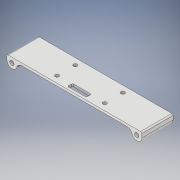
# Autodesk Inventor part: US Halterung hinten leicht
Saved by Autodesk Inventor 2018 (Build 220112000, 112)
## iProperties
Created: 2019-03-05
Part Number: US Halterung hinten leicht
Material: ABS-Kunststoff
Document SubType Name: Modeling
Designer: RedBots
Density: 0.732517 g/cm^3
Appearance: Glatt - weiß
Mass: 4 g
Surface Area: 43.527 cm^2
Volume: 5.46063 cm^3
Author: RedBots
Autodesk Inventor part; units mm, degrees
ref_plane "YZ Plane" through (0, 0, 0) normal (1, 0, 0) x (0, 1, 0)
ref_plane "XZ Plane" through (0, 0, 0) normal (0, 1, 0) x (-1, 0, 0)
ref_plane "XY Plane" through (0, 0, 0) normal (0, 0, 1) x (1, 0, 0)
sketch "Skizze1" plane through (0, 0, 0) normal (0, 0, 1) x (1, 0, 0)
  line L0 (0, 0) -> (108, 0)
  line L1 (108, 0) -> (108, 25)
  line L2 (108, 25) -> (0, 25)
  line L3 (0, 25) -> (0, 0)
  dimension "d5" = 108
  dimension "d6" = 25
  constraints: 8 end point, 2 parallel, 1 horizontal, 1 perpendicular
  measures "d5" distance of L1.end L2.end
  measures "d6" distance of L0.end L1.end
extrude "Extrusion1" add sketch "Skizze1" along normal blind 2
sketch "Skizze3" plane through (0, 25, 0) normal (0, 1, 0) x (1, 0, 0)
  circle A0 centre (4, 2) radius 1.75
  circle A1 centre (104, 2) radius 1.75
  line L0 (4, 2) -> (104, 2) construction
  line L1 (0, 0) -> (108, 0) construction
  line L2 (54, 0) -> (54, 2) construction
  line L3 (0, 0) -> (8, 0)
  line L4 (108, 0) -> (100, 0)
  line L5 (0, 0) -> (0, 2)
  line L6 (8, 2) -> (8, 0)
  line L7 (100, 2) -> (100, 0)
  line L8 (108, 0) -> (108, 2)
  arc A2 (8, 2) -> (0, 2) centre (4, 2) ccw
  arc A3 (108, 2) -> (100, 2) centre (104, 2) ccw
  dimension "d2" = 100
  dimension "d3" = 3.5
  dimension "d4" = 2
  constraints: 16 end point, 5 parallel, 4 centre point, 4 point on circle, 3 horizontal, 3 vertical, 2 coincident, 2 midpoint, 2 point on line, 1 equal radius
  measures "d2" distance of L0.start L0.end
  measures "d3" diameter of A0
  measures "d4" distance of L2.start L2.end
extrude "Extrusion2" add sketch "Skizze3" against normal up to surface (25 mm away)
sketch "Skizze4" plane through (0, 0, 2) normal (0, 0, 1) x (1, 0, 0)
  line L0 (34.95, 5.261) -> (73.05, 5.261) construction
  line L1 (73.05, 5.261) -> (73.05, 19.739) construction
  line L2 (73.05, 19.739) -> (34.95, 19.739) construction
  line L3 (34.95, 19.739) -> (34.95, 5.261) construction
  line L4 (108, 25) -> (0, 25) construction
  line L5 (54, 25) -> (54, 0) construction
  line L6 (0, 0) -> (108, 0) construction
  line L7 (0, 25) -> (0, 0) construction
  line L8 (0, 12.5) -> (108, 12.5) construction
  line L9 (108, 0) -> (108, 25) construction
  circle A0 centre (73.05, 19.739) radius 1.5
  circle A1 centre (34.95, 5.261) radius 1.5
  circle A2 centre (34.95, 19.739) radius 1.5
  circle A3 centre (73.05, 5.261) radius 1.5
  point P0 (54, 19.739)
  point P1 (73.05, 12.5)
  dimension "d12" = 38.1
  dimension "d13" = 14.478
  dimension "d14" = 3
  constraints: 12 end point, 6 midpoint, 4 centre point, 4 coincident, 3 equal radius, 2 parallel, 2 point on line, 1 horizontal, 1 perpendicular
  measures "d12" distance of L1.end L2.end
  measures "d13" distance between parallel lines of L0 L2
  measures "d14" diameter of A0
extrude "Extrusion3" cut sketch "Skizze4" against normal blind 8
sketch "Skizze5" plane through (0, 0, 2) normal (0, 0, 1) x (1, 0, 0)
  line L0 (44.09, 22.4949) -> (0.91, 22.4949) construction
  line L1 (0.91, 22.4949) -> (0.91, 2.5051) construction
  line L2 (0.91, 2.5051) -> (44.09, 2.5051) construction
  line L3 (44.09, 2.5051) -> (44.09, 22.4949) construction
  line L4 (108, 25) -> (0, 25) construction
  line L5 (54, 25) -> (54, 0) construction
  line L6 (0, 0) -> (108, 0) construction
  line L7 (108, 0) -> (108, 25) construction
  line L8 (108, 12.5) -> (0, 12.5) construction
  line L9 (0, 25) -> (0, 0) construction
  line L10 (46.5, 6.0051) -> (61.5, 6.0051)
  line L11 (61.5, 6.0051) -> (61.5, 2.0051)
  line L12 (61.5, 2.0051) -> (46.5, 2.0051)
  line L13 (46.5, 2.0051) -> (46.5, 6.0051)
  point P0 (0.91, 12.5)
  point P1 (54, 6.0051)
  dimension "d17" = 43.18
  dimension "d18" = 19.9898
  dimension "d19" = 15
  dimension "d20" = 4
  dimension "d27" = 0.5
  constraints: 20 end point, 6 midpoint, 4 parallel, 2 horizontal, 2 perpendicular, 2 point on line
  measures "d17" distance of L0.start L0.end
  measures "d18" distance of L0.end L1.end
  measures "d19" distance of L11.end L12.end
  measures "d20" distance of L10.end L11.end
  measures "d27" distance between parallel lines of L2 L12
extrude "Extrusion4" cut sketch "Skizze5" against normal up to next
fillet "Rundung1" radius 1 4 edges at (46.5, 6.0051, 1) (61.5, 6.0051, 1) (61.5, 2.0051, 1) (46.5, 2.0051, 1)
fillet "Rundung2" radius 4 2 edges at (8, 12.5, 0) (100, 12.5, 0)
fillet "Rundung3" radius 1 2 edges at (0, 12.5, 2) (108, 12.5, 2)
